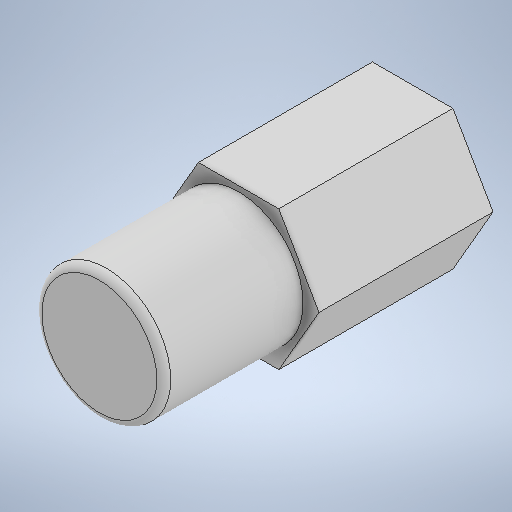
# Autodesk Inventor part: hex_shaft
Saved by Autodesk Inventor 2025 (Build 290162000, 162)
## iProperties
Created: 2024-06-17
Part Number: hex_shaft
Material: Generic
Document SubType Name: Modeling
Designer: Pintu
Density: 1 g/cm^3
Appearance: Default
Author: Pintu
Autodesk Inventor part; units mm, degrees
ref_plane "YZ Plane" through (0, 0, 0) normal (1, 0, 0) x (0, 1, 0)
ref_plane "XZ Plane" through (0, 0, 0) normal (0, 1, 0) x (-1, 0, 0)
ref_plane "XY Plane" through (0, 0, 0) normal (0, 0, 1) x (1, 0, 0)
sketch "Sketch1" plane through (0, 0, 0) normal (0, 0, 1) x (1, 0, 0)
  line L0 (2.3094, -4) -> (-2.3094, -4)
  line L1 (-2.3094, -4) -> (-4.6188, 0)
  line L2 (-4.6188, 0) -> (-2.3094, 4)
  line L3 (-2.3094, 4) -> (2.3094, 4)
  line L4 (2.3094, 4) -> (4.6188, 0)
  line L5 (4.6188, 0) -> (2.3094, -4)
  point P0 (0, 0)
  point P1 (0, 0)
  dimension "d0" = 8
  constraints: 12 end point, 1 coincident, 1 horizontal, 13 other
  measures "d0" distance between parallel lines of L0 L3
extrude "Extrusion1" add sketch "Sketch1" along normal blind 10
sketch "Sketch2" plane through (0, 0, 10) normal (0, 0, 1) x (1, 0, 0)
  circle A0 centre (0, 0) radius 3.7
  dimension "d3" = 7.4
  constraints: 1 centre point, 1 coincident
  measures "d3" diameter of A0
extrude "Extrusion2" add sketch "Sketch2" along normal blind 8
fillet "Fillet1" radius 0.4 1 edges at (-3.7, 0, 18)
body "Solid1"
